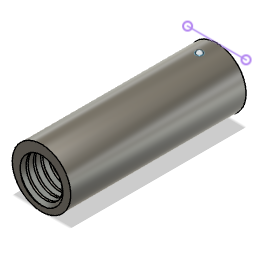
gasChargingBombLid v4 (Autodesk Fusion 360 design; units mm, degrees)
Autodesk Fusion 360 part; units mm, degrees
sketch "Skizze1" plane through (0, 0, 0) normal (0, 0, 1) x (1, 0, 0)
  circle A0 centre (0, 0) radius 5
  dimension "d1" = 10
  constraint coincident A0.centre origin
  measures "d1" diameter of A0
extrude "Extrusion1" add sketch "Skizze1" along normal blind 30
ref_plane "Arbeitsebene1" through (0, 5, 2.1001) normal (0, 1, 0) x (1, 0, 0)
sketch "Skizze3" plane through (0, 5, 2.1001) normal (0, 1, 0) x (1, 0, 0)
  line L0 (-5, 2.1001) -> (5, 2.1001)
  circle A0 centre (0, -0.8999) radius 0.5
  dimension "d16" = 1
  dimension "d17" = 3
  measures "d16" diameter of A0
  measures "d17" distance of L0 A0.centre
sketch "Skizze4" plane through (0, 0, 30) normal (0, 0, 1) x (1, 0, 0)
  circle A0 centre (0, 0) radius 5
  circle A1 centre (0, 0) radius 3.9
  dimension "d12" = 7.8
  constraint concentric A0 A1
  measures "d12" diameter of A1
extrude "Extrusion3" cut sketch "Skizze4" against normal blind 28 contours A1
extrude "Extrusion4" cut sketch "Skizze3" against normal through all
thread "Gewinde2" "ISO Metric profile 8.0 M8x1.25 6H" major diameter 8.17 minor diameter 6.7795 pitch 1.25 angle 60 modelled right hand crest width 0.343 on face at (3.8806, -0.3883, 11.3333) crest through (3.3898, 0, 29.6875)
